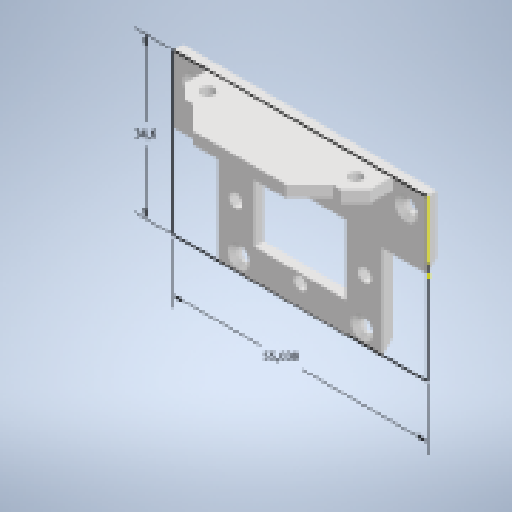
# Autodesk Inventor part: bloco_aquecimento
Saved by Autodesk Inventor 2025.1 (Build 291241000, 241)
## iProperties
Created: 2024-03-21
Part Number: bloco_aquecimento
Material: Genérico
Document SubType Name: Modeling
Designer: joaov
Density: 1 g/cm^3
Appearance: Padrão
Author: joaov
Autodesk Inventor part; units mm, degrees
ref_plane "YZ Plane" through (0, 0, 0) normal (1, 0, 0) x (0, 1, 0)
ref_plane "XZ Plane" through (0, 0, 0) normal (0, 1, 0) x (-1, 0, 0)
ref_plane "XY Plane" through (0, 0, 0) normal (0, 0, 1) x (1, 0, 0)
sketch "Esboço1" plane through (0, 0, 0) normal (0, 0, 1) x (1, 0, 0)
  line L0 (0, 0) -> (0, 15.2)
  line L1 (0, 15.2) -> (-55.362, 15.2)
  line L2 (-55.362, 15.2) -> (-55.362, 0)
  line L3 (-55.362, 0) -> (-45.681, 0)
  line L4 (-45.681, 0) -> (-45.681, -20.1)
  line L5 (-45.681, -20.1) -> (-9.681, -20.1)
  line L6 (-9.681, -20.1) -> (-9.681, 0)
  line L7 (-9.681, 0) -> (0, 0)
  line L8 (-27.681, 15.2) -> (-27.681, 10.2)
  line L9 (-27.681, -20.1) -> (-27.681, -16.9)
  circle A0 centre (-40.981, -16.9) radius 1.4
  circle A1 centre (-50.662, 10.2) radius 1.4
  circle A2 centre (-14.381, -16.9) radius 1.4
  circle A3 centre (-4.7, 10.2) radius 1.4
  dimension "d0" = 15.2
  dimension "d1" = 55.362
  dimension "d2" = 15.2
  dimension "d4" = 20.1
  dimension "d5" = 36
  dimension "d6" = 20.1
  dimension "d7" = 5
  dimension "d8" = 3.2
  dimension "d290" = 2.8
  dimension "d291" = 2.8
  dimension "d292" = 2.8
  dimension "d293" = 2.8
  constraints: 20 end point, 4 centre point, 4 perpendicular, 3 vertical, 2 midpoint, 1 horizontal, 1 point on line
  measures "d0" distance of L0.start L0.end
  measures "d1" distance of L0.end L1.end
  measures "d2" distance of L1.end L2.end
  measures "d4" distance of L3.end L4.end
  measures "d5" distance of L4.end L5.end
  measures "d6" distance of L5.end L6.end
  measures "d7" distance of L8.start L8.end
  measures "d8" distance of L9.start L9.end
  measures "d290" diameter of A0
  measures "d291" diameter of A1
  measures "d292" diameter of A2
  measures "d293" diameter of A3
extrude "Extrusão1" add sketch "Esboço1" along normal blind 4.5
sketch "Esboço15" plane through (0, 0, 4.5) normal (0, 0, 1) x (1, 0, 0)
  line L0 (0, 15.2) -> (-55.362, 15.2) projected
  line L1 (-45.681, -20.1) -> (-9.681, -20.1) projected
  line L2 (-27.681, 15.2) -> (-7.681, 15.2)
  line L3 (-27.681, 15.2) -> (-47.681, 15.2)
  line L4 (-47.681, 15.2) -> (-47.681, 12.2)
  line L5 (-47.681, 12.2) -> (-7.681, 12.2)
  line L6 (-7.681, 12.2) -> (-7.681, 15.2)
  line L7 (-27.681, 12.2) -> (-27.681, 1.7)
  point P0 (0, 0)
  point P1 (-55.362, 0)
  point P2 (-47.681, 0)
  dimension "d146" = 20
  dimension "d147" = 20
  dimension "d190" = 3
  dimension "d198" = 10.5
  constraints: 12 end point, 3 point on line, 2 midpoint, 2 vertical
  measures "d146" distance of L2.start L2.end
  measures "d147" distance of L2.start L3.end
  measures "d190" distance of L3.end L4.end
  measures "d198" distance of L7.start L7.end
extrude "Extrusão10" add sketch "Esboço15" along normal blind 8
sketch "Esboço18" plane through (0, 0, 4.5) normal (0, 0, 1) x (1, 0, 0)
  line L0 (-42.181, 9.2) -> (-45.181, 9.2) projected
  line L1 (0, 15.2) -> (-55.362, 15.2) projected
  circle A0 centre (-27.681, -15.1) radius 1.4
  line L2 (-27.681, 0) -> (-37.681, 0)
  line L3 (-27.681, -13.3) -> (-37.681, -13.3)
  line L4 (-37.681, -13.3) -> (-37.681, 0)
  line L5 (-37.681, 0) -> (-17.681, 0)
  line L6 (-17.681, 0) -> (-17.681, -13.3)
  line L7 (-17.681, -13.3) -> (-37.681, -13.3)
  line L8 (-37.681, -13.3) -> (-37.681, 0)
  line L9 (-7.681, 12.2) -> (-47.681, 12.2) projected
  line L10 (-27.681, 12.2) -> (-27.681, 1.7)
  line L11 (-27.681, 0) -> (-27.681, 1.7)
  line L12 (-37.681, 0) -> (-17.681, 0)
  line L13 (-17.681, 0) -> (-17.681, 1.7)
  line L14 (-17.681, 1.7) -> (-37.681, 1.7)
  line L15 (-37.681, 1.7) -> (-37.681, 0)
  point P0 (0, 0)
  point P1 (-35.681, 15.2)
  point P2 (-19.681, 15.2)
  dimension "d224" = 2.8
  dimension "d227" = 20
  dimension "d232" = 10.5
  dimension "d240" = 15
  dimension "d241" = 20
  constraints: 26 end point, 4 parallel, 4 perpendicular, 2 horizontal, 1 centre point, 1 midpoint, 1 vertical
  measures "d224" diameter of A0
  measures "d227" distance of L6.end L7.end
  measures "d232" distance of L10.start L10.end
  measures "d240" distance of L6.end L13.end
  measures "d241" distance of L13.end L14.end
extrude "Extrusão13" cut sketch "Esboço18" against normal blind 10
sketch "Esboço20" plane through (-47.681, 12.2, 4.5) normal (0, -1, 0) x (1, 0, 0)
  line L0 (40, 0) -> (0, 0)
  line L1 (0, 0) -> (40, 0)
  line L2 (0, 0) -> (0, 8)
  line L3 (0, 0) -> (2, 0)
  line L4 (2, 0) -> (38, 0)
  line L5 (0, 8) -> (8, 8)
  line L6 (8, 8) -> (8, 0)
  line L7 (8, 0) -> (0, 0)
  line L8 (0, 0) -> (0, 8)
  line L9 (40, 8) -> (0, 8)
  line L10 (40, 8) -> (32, 8)
  line L11 (32, 8) -> (32, 0)
  line L12 (32, 0) -> (40, 0)
  line L13 (40, 0) -> (40, 8)
  line L14 (8, 8) -> (32, 8)
  line L15 (32, 8) -> (32, 0)
  line L16 (32, 0) -> (8, 0)
  line L17 (8, 0) -> (8, 8)
  line L18 (40, 8) -> (0, 8) projected
  line L19 (0, 8) -> (0, 6.5641)
  line L20 (0, 0) -> (0, 8) projected
  circle A0 centre (4, 4) radius 1.4
  circle A1 centre (36, 4) radius 1.4
  point P0 (47.681, -4.5)
  point P1 (47.681, -2.5)
  point P2 (0, 4)
  point P3 (72.5443, 10.7201)
  point P4 (72.5443, 18.7201)
  point P5 (48.5443, 10.7201)
  dimension "d194" = 8
  dimension "d195" = 8
  dimension "d230" = 2.8
  dimension "d231" = 2.8
  constraints: 38 end point, 7 equal length, 4 point on line, 3 horizontal, 3 perpendicular, 2 centre point, 1 midpoint
  measures "d194" distance of L6.end L7.end
  measures "d195" distance of L12.end L11.end
  measures "d230" diameter of A0
  measures "d231" diameter of A1
extrude "Extrusão14" cut sketch "Esboço20" along normal blind 15 and the other way blind 3 contours A0 | A1
sketch "Esboço21" plane through (0, 0, 4.5) normal (0, 0, 1) x (1, 0, 0)
  line L0 (-55.362, 15.2) -> (-55.362, 0) projected
  line L1 (-55.362, 15.2) -> (-55.262, 15.2)
  line L2 (-47.681, 15.2) -> (-55.362, 15.2) projected
  line L3 (0, 15.2) -> (-55.362, 15.2) projected
  line L4 (0, 15.2) -> (-0.1, 15.2)
  line L5 (-9.681, 0) -> (0, 0) projected
  line L6 (0, 0) -> (-0.1, 0)
  line L7 (-9.681, -20.1) -> (-9.681, 0) projected
  line L8 (-9.681, -20.1) -> (-9.781, -20.1)
  line L9 (-45.681, -20.1) -> (-9.681, -20.1) projected
  line L10 (-45.681, -20.1) -> (-45.581, -20.1)
  line L11 (-45.581, -20.1) -> (-45.681, -20.1)
  line L12 (-45.681, 0) -> (-45.681, -20.1) projected
  line L13 (-55.362, 0) -> (-45.681, 0) projected
  line L14 (-55.362, 0) -> (-55.262, 0)
  line L15 (-55.262, 0.1) -> (-45.581, 0.1)
  line L16 (-45.581, 0.1) -> (-45.581, -20)
  line L17 (-45.581, -20) -> (-9.781, -20)
  line L18 (-9.781, -20) -> (-9.781, 0)
  line L19 (-9.781, 0) -> (-9.781, 0.1)
  line L20 (-9.781, 0.1) -> (-9.681, 0.1)
  line L21 (-9.781, 0.1) -> (-9.681, 0.1)
  line L22 (-9.681, 0.1) -> (-0.1, 0.1)
  line L23 (0, 0) -> (0, 15.2) projected
  line L24 (-0.1, 0.1) -> (-0.1, 15.1)
  line L25 (-0.1, 15.1) -> (-55.262, 15.1)
  line L26 (-55.262, 15.1) -> (-55.262, 0.1)
  line L27 (-55.362, 15.2) -> (-55.362, 0)
  line L28 (-55.362, 0) -> (-45.681, 0)
  line L29 (-45.681, 0) -> (-45.681, -20.1)
  line L30 (-45.681, -20.1) -> (-9.681, -20.1)
  line L31 (-9.681, -20.1) -> (-9.681, 0)
  line L32 (-9.681, 0) -> (0, 0)
  line L33 (0, 0) -> (0, 15.2)
  line L34 (0, 15.2) -> (-55.362, 15.2)
  dimension "d203" = 0.1
  dimension "d204" = 0.1
  constraints: 52 end point, 6 perpendicular, 6 point on line, 4 equal length, 2 vertical
  measures "d203" distance of L0.start L1.end
  measures "d204" distance of L1.end L25.end
extrude "Extrusão15" cut sketch "Esboço21" along normal mid plane 20.5
sketch "Esboço22" plane through (0, 0, 4.5) normal (0, 0, 1) x (1, 0, 0)
  circle A0 centre (-41.631, -6.65) radius 1.4
  circle A1 centre (-13.731, -6.65) radius 1.4
  line L0 (-37.681, -13.3) -> (-37.681, 1.7) projected
  point P0 (0, 0)
  point P1 (-17.681, 0)
  dimension "d236" = 2.8
  dimension "d237" = 2.8
  dimension "d242" = 3.95
  constraints: 2 centre point
  measures "d236" diameter of A0
  measures "d237" diameter of A1
  measures "d242" distance from line of L0 A0.centre
extrude "Extrusão16" cut sketch "Esboço22" against normal through all
sketch "Esboço23" plane through (0, 0, 12.5) normal (0, 0, 1) x (1, 0, 0)
  line L0 (-37.681, -13.3) -> (-37.681, 1.7) projected
  line L1 (-7.681, 15.1) -> (-47.681, 15.1) projected
  line L2 (-37.681, 1.7) -> (-17.681, 1.7) projected
  line L3 (-37.681, 15.1) -> (-17.681, 15.1)
  line L4 (-7.681, 12.2) -> (-47.681, 12.2) projected
  line L5 (-37.681, 12.2) -> (-17.681, 12.2)
  line L6 (-37.681, 15.1) -> (-37.681, 12.2)
  line L7 (-17.681, 15.1) -> (-17.681, 12.2)
  point P0 (0, 0)
  constraints: 8 end point, 4 point on line, 2 perpendicular
extrude "Extrusão17" add sketch "Esboço23" along normal blind 5
chamfer "Chanfro3" distance 5 angle 45 2 edges at (-37.681, 13.65, 12.5) (-17.681, 13.65, 12.5)
chamfer "Chanfro4" distance 3 angle 45 2 edges at (-47.681, 13.65, 12.5) (-7.681, 13.65, 12.5)
sketch "Esboço24" plane through (-9.781, -20, 4.5) normal (1, 0, 0) x (0, 0, -1)
  line L0 (2.5, 0.2) -> (4.5, 0.2)
  line L1 (3.4293, 1.2707) -> (4.5, 2.3414)
  line L2 (3.4293, 1.2707) -> (2.3586, 0.2)
  line L3 (4.5, 2.3414) -> (4.5, 0.2)
  line L4 (2.3586, 0.2) -> (4.5, 0.2)
  line L5 (4.5, 2.1414) -> (4.5, 2.3414)
  line L6 (0, 0) -> (0, 20.1) projected
  line L7 (4.5, 0) -> (0, 0)
  line L8 (0, 0) -> (0, 0.2)
  line L9 (0, 0.2) -> (4.5, 0.2)
  line L10 (4.5, 0.2) -> (4.5, 0)
  point P0 (4.5, 20)
  point P1 (4.5, 0.2)
  point P2 (2.3586, 0.2)
  dimension "d270" = 0.2
  constraints: 20 end point, 2 horizontal, 2 parallel, 1 perpendicular, 1 point on line
  measures "d270" distance of L5.start L5.end
extrude "Extrusão18" cut sketch "Esboço24" against normal through all
sketch "Esboço25" plane through (-0.1, 0.1, 4.5) normal (1, 0, 0) x (0, 0, -1)
  line L0 (3.4, 1.2) -> (4.5, 2.3)
  line L1 (3.4, 1.2) -> (2.4, 0.2)
  line L2 (2.4, 0.2) -> (4.5, 0.2)
  line L3 (4.5, 0.2) -> (4.5, 2.3)
  line L4 (4.5, 2.3) -> (3.95, 2.3)
  line L5 (4.899, 0.2) -> (-0.488, 0.2)
  line L6 (-0.488, 0.2) -> (-0.488, 0)
  line L7 (-0.488, 0) -> (4.899, 0)
  line L8 (4.899, 0) -> (4.899, 0.2)
  point P0 (4.5, 0)
  point P1 (2.4, 0.2)
  constraints: 18 end point, 2 horizontal, 2 parallel, 2 perpendicular, 1 point on line
extrude "Extrusão19" cut sketch "Esboço25" against normal blind 9.681
sketch "Esboço26" plane through (-55.262, 0.1, 4.5) normal (-1, 0, 0) x (0, 0, 1)
  line L0 (-4.5, 2.3) -> (-2.4, 0.2)
  line L1 (-4.5, 0.2) -> (-2.4, 0.2)
  line L2 (-4.5, 0.2) -> (-2.4, 0.2)
  line L3 (-4.5, 2.3) -> (-4.5, 0.2)
  line L4 (-4.5, 0) -> (-4.5, -17.7586) projected
  line L5 (-4.5, 0) -> (-4.5, 15) projected
  line L6 (-4.5, 2.3) -> (-4.3, 2.3)
  line L7 (-4.7094, 0.2) -> (0.2738, 0.2)
  line L8 (0.2738, 0.2) -> (0.2738, 0)
  line L9 (0.2738, 0) -> (-4.7094, 0)
  line L10 (-4.7094, 0) -> (-4.7094, 0.2)
  point P0 (-2.4, 0.2)
  constraints: 18 end point, 3 horizontal, 2 collinear, 2 parallel, 1 perpendicular, 1 point on line
extrude "Extrusão20" cut sketch "Esboço26" against normal blind 9.681
sketch "Esboço27" plane through (0, 0, 17.5) normal (0, 0, 1) x (1, 0, 0)
  line L0 (-55.262, 15.1) -> (-0.1, 15.1) projected
  line L1 (-55.262, 15.1) -> (-55.262, 14.8)
  line L2 (-55.262, 15.1) -> (-55.262, 0.3) projected
  line L3 (-55.262, 14.8) -> (-0.1, 14.8)
  line L4 (-0.1, 0.3) -> (-0.1, 15.1) projected
  line L5 (-0.1, 14.8) -> (-55.262, 14.8)
  line L6 (-55.262, 14.8) -> (-55.262, 15.7059)
  line L7 (-55.262, 15.7059) -> (-0.1, 15.7059)
  line L8 (-0.1, 15.7059) -> (-0.1, 14.8)
  point P0 (0, 0)
  point P1 (-0.1, 15.1)
  dimension "d273" = 0.3
  dimension "d274" = 90
  constraints: 12 end point, 2 parallel, 2 point on line, 1 horizontal, 1 perpendicular
  measures "d273" distance of L0.start L1.end
  measures "d274" angle of L3 L1
extrude "Extrusão21" cut sketch "Esboço27" against normal through all
sketch "Esboço28" plane through (-37.681, 14.8, 17.5) normal (0, 1, 0) x (1, 0, 0)
  line L0 (-17.581, 17.5) -> (37.581, 17.5) projected
  line L1 (-17.581, 17.5) -> (-17.481, 17.5)
  line L2 (-17.481, 17.5) -> (-17.481, 12.5734)
  line L3 (-17.481, 17.5) -> (-17.7304, 17.5)
  line L4 (-17.7304, 17.5) -> (-17.7304, 12.8429)
  line L5 (-17.7304, 12.8429) -> (-17.481, 12.8429)
  line L6 (-17.481, 12.8429) -> (-17.481, 17.5)
  line L7 (0, 17.5) -> (20, 17.5) projected
  line L8 (10, 17.5) -> (10, 11.5745)
  line L9 (37.581, 17.5) -> (37.481, 17.5)
  line L10 (37.481, 17.5) -> (37.481, 12.5734)
  line L11 (37.481, 17.5) -> (37.7304, 17.5)
  line L12 (37.7304, 17.5) -> (37.7304, 12.8429)
  line L13 (37.7304, 12.8429) -> (37.481, 12.8429)
  line L14 (37.481, 12.8429) -> (37.481, 17.5)
  point P0 (37.681, 17.5)
  point P1 (-17.481, 12.8429)
  constraints: 26 end point, 5 symmetric about line, 2 parallel, 2 perpendicular, 1 horizontal, 1 midpoint, 1 point on line, 1 vertical
extrude "Extrusão22" cut sketch "Esboço28" against normal through all
sketch "Esboço29" plane through (-9.781, -19.8, 2.1414) normal (0, -1, 0) x (1, 0, 0)
  line L0 (0, 0) -> (0, -2.1414) projected
  line L1 (0, 0) -> (-0.1, 0)
  line L2 (0, 0) -> (-35.8, 0) projected
  line L3 (-0.1, 0) -> (-0.1, -2.4621)
  line L4 (-0.1, 0) -> (-0.1, 2.728)
  line L5 (-0.1, 2.728) -> (0.1398, 2.728)
  line L6 (0.1398, 2.728) -> (0.1398, -2.4621)
  line L7 (0.1398, -2.4621) -> (-0.1, -2.4621)
  line L8 (-0.1, -2.4621) -> (-0.1, 2.728)
  line L9 (-17.9, 0) -> (-17.9, -4.1402)
  line L10 (-35.8, 0) -> (-35.8, -2.1414)
  line L11 (-35.8, 0) -> (-35.7, 0)
  line L12 (-35.7, 0) -> (-35.7, -2.4621)
  line L13 (-35.7, 0) -> (-35.7, 2.728)
  line L14 (-35.7, 2.728) -> (-35.9398, 2.728)
  line L15 (-35.9398, 2.728) -> (-35.9398, -2.4621)
  line L16 (-35.9398, -2.4621) -> (-35.7, -2.4621)
  line L17 (-35.7, -2.4621) -> (-35.7, 2.728)
  point P0 (9.781, -2.1414)
  point P1 (-0.1, -2.4621)
  dimension "d280" = 0.1
  constraints: 32 end point, 7 symmetric about line, 3 vertical, 2 parallel, 1 horizontal, 1 midpoint, 1 perpendicular, 1 point on line
  measures "d280" distance of L0.start L1.end
extrude "Extrusão23" cut sketch "Esboço29" against normal blind 20.1
sketch "Esboço30" plane through (-45.581, 0.3, 0) normal (-1, 0, 0) x (0, 0, 1)
  line L0 (0, 2.1) -> (2.1, 0) projected
  line L1 (2.1, 0) -> (0, 2.1)
  line L2 (0, 0) -> (0, 2.1) projected
  line L3 (0, 2.1) -> (0, 0)
  line L4 (0, 0) -> (2.1, 0)
  point P0 (0, -0.3)
  constraints: 6 end point, 2 collinear, 1 perpendicular
extrude "Extrusão24" cut sketch "Esboço30" against normal blind 0.1
sketch "Esboço31" plane through (-9.781, 0.3, 0) normal (1, 0, 0) x (0, 0, -1)
  line L0 (-2.1, 0) -> (0, 2.1) projected
  line L1 (0, 2.1) -> (-2.1, 0)
  line L2 (0, 0) -> (-4.5, 0) projected
  line L3 (-2.1, 0) -> (0, 0)
  line L4 (0, 0) -> (0, 2.1)
  point P0 (0, -0.3)
  constraints: 6 end point, 2 collinear, 1 perpendicular
extrude "Extrusão25" cut sketch "Esboço31" against normal blind 0.1
sketch "Esboço33" plane through (0, 0, 4.5) normal (0, 0, 1) x (1, 0, 0)
  line L0 (-0.2, 14.8) -> (-0.2, 2.4) projected
  line L1 (-0.2, 14.8) -> (-55.2376, 14.8)
  line L2 (-55.2376, 14.8) -> (-55.2376, -19.8)
  line L3 (-55.2376, -19.8) -> (-0.2, -19.8)
  line L4 (-0.2, -19.8) -> (-0.2, 14.8)
  point P0 (0, 0)
  dimension "d288" = 34.6
  dimension "d289" = 55.0376
  constraints: 8 end point, 2 parallel, 1 horizontal, 1 perpendicular
  measures "d288" distance of L1.end L2.end
  measures "d289" distance of L2.end L3.end
chamfer "Chanfro5" distance 1 angle 45 4 edges at (-42.381, -16.9, 4.5) (-52.062, 10.2, 4.5) (-15.781, -16.9, 4.5) (-6.1, 10.2, 4.5)
sketch "Esboço34" plane through (-0.2, 14.8, 4.5) normal (1, 0, 0) x (0, 0, -1)
  line L0 (0, -34.6) -> (2.1414, -32.4586)
  line L1 (2.1414, -32.4586) -> (2.1414, -34.6)
  line L2 (2.1414, -34.6) -> (0, -34.6)
  line L3 (2.1414, -34.6) -> (5.2447, -34.6)
  line L4 (5.2447, -34.6) -> (5.2447, 1.8911)
  line L5 (5.2447, 1.8911) -> (2.1414, 1.8911)
  line L6 (2.1414, 1.8911) -> (2.1414, -34.6)
  point P0 (4.5, -14.8)
  constraints: 14 end point, 2 parallel, 2 perpendicular, 1 horizontal, 1 vertical
extrude "Extrusão26" cut sketch "Esboço34" against normal through all
sketch "Esboço35" plane through (-0.2, 0.3, 4.5) normal (1, 0, 0) x (0, 0, -1)
  line L0 (2.1414, 2.1414) -> (0, 0)
  line L1 (0, 0) -> (2.1414, 0)
  line L2 (2.1414, 0) -> (2.1414, 2.1414)
  line L3 (2.1414, 0) -> (0, 0) projected
  point P0 (4.5, -0.3)
  constraints: 6 end point, 1 perpendicular
extrude "Extrusão27" cut sketch "Esboço35" against normal blind 9.681
sketch "Esboço36" plane through (-55.162, 0.3, 4.5) normal (-1, 0, 0) x (0, 0, 1)
  line L0 (0, -20.1) -> (-2.1414, -17.9586) projected
  line L1 (0, 0) -> (-2.1414, 2.1414)
  line L2 (-2.1414, 2.1414) -> (-2.1414, 0)
  line L3 (-2.1414, 0) -> (0, 0)
  point P0 (0, 0)
  point P1 (-2.1414, 0)
  constraints: 6 end point, 1 perpendicular
extrude "Extrusão28" cut sketch "Esboço36" against normal blind 9.681
sketch "Esboço37" plane through (-0.2, 14.8, 4.5) normal (1, 0, 0) x (0, 0, -1)
  line L0 (2.1414, -12.3586) -> (2.1414, 0) projected
  line L1 (2.1414, 0) -> (0, 0) projected
  line L2 (2.1414, 0) -> (0, 0)
  point P0 (4.5, -14.8)
  dimension "d305" = 2.1414
  constraints: 2 end point, 1 collinear
  measures "d305" distance of L0.end L1.end
